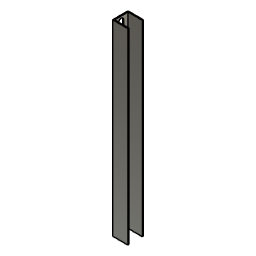
strut v1 (Autodesk Fusion 360 design; units mm, degrees)
Autodesk Fusion 360 part; units mm, degrees
sketch "Sketch1" plane through (0, 0, 0) normal (0, 0, 1) x (1, 0, 0)
  line L0 (20.5, 20.5) -> (-20.5, 20.5)
  line L1 (-20.5, 20.5) -> (-20.5, -20.5)
  line L2 (-20.5, -20.5) -> (20.5, -20.5)
  line L3 (20.5, -20.5) -> (20.5, 20.5)
  line L4 (20.5, 20.5) -> (-20.5, -20.5) construction
  line L5 (-20.5, 20.5) -> (20.5, -20.5) construction
  line L6 (-18, -18) -> (18, -18)
  line L7 (18, -18) -> (18, 18)
  line L8 (18, 18) -> (-18, 18)
  line L9 (-18, 18) -> (-18, -18)
  line L10 (18, 18) -> (20.5, 18)
  line L11 (20.5, 18) -> (20.5, -18)
  line L12 (20.5, -18) -> (18, -18)
  line L13 (18, -18) -> (18, 18)
  dimension "d1" = 41
  dimension "d2" = 41
  dimension "d3" = -2.5
  constraint horizontal L0
  constraint perpendicular L0 L1
  constraint parallel L0 L2
  constraint parallel L1 L3
  constraint coincident L4 origin
  constraint coincident L5 origin
  constraint horizontal L10
  constraint vertical L11
  constraint horizontal L12
  constraint vertical L13
  constraint coincident L3 L11.end
  measures "d1" distance of L1.end L2.end
  measures "d2" distance of L0.end L1.end
extrude "Extrude1" add sketch "Sketch1" along normal blind 500 contours L0 L1 L2 L3 L6 L8 L9 L10 L12
sketch "Sketch2" plane through (-20.5, 0, 0) normal (-1, 0, 0) x (0, -1, 0)
  line L0 (-20.5, 0) -> (20.5, 0)
  line L1 (20.5, 0) -> (20.5, 500)
  line L2 (20.5, 500) -> (-20.5, 500)
  line L3 (-20.5, 500) -> (-20.5, 0)
  line L4 (0, 500) -> (0, 495)
  line L5 (-6.5, 488.5) -> (-6.5, 461.5)
  line L6 (6.5, 488.5) -> (6.5, 461.5)
  arc A0 (0, 495) -> (-6.5, 488.5) centre (0, 488.5) ccw
  arc A1 (-6.5, 461.5) -> (0, 455) centre (0, 461.5) ccw
  arc A2 (0, 455) -> (6.5, 461.5) centre (0, 461.5) ccw
  arc A3 (6.5, 488.5) -> (0, 495) centre (0, 488.5) ccw
  line L7 (0, 455) -> (0, 432.5)
  line L8 (-6.5, 426) -> (-6.5, 399)
  arc A4 (0, 432.5) -> (-6.5, 426) centre (0, 426) ccw
  arc A5 (6.5, 426) -> (0, 432.5) centre (0, 426) ccw
  line L9 (6.5, 426) -> (6.5, 399)
  arc A6 (0, 392.5) -> (6.5, 399) centre (0, 399) ccw
  arc A7 (-6.5, 399) -> (0, 392.5) centre (0, 399) ccw
  line L10 (-6.5, 363.5) -> (-6.5, 336.5)
  arc A8 (0, 370) -> (-6.5, 363.5) centre (0, 363.5) ccw
  arc A9 (6.5, 363.5) -> (0, 370) centre (0, 363.5) ccw
  line L11 (6.5, 363.5) -> (6.5, 336.5)
  arc A10 (0, 330) -> (6.5, 336.5) centre (0, 336.5) ccw
  arc A11 (-6.5, 336.5) -> (0, 330) centre (0, 336.5) ccw
  line L12 (-6.5, 301) -> (-6.5, 274)
  arc A12 (0, 307.5) -> (-6.5, 301) centre (0, 301) ccw
  arc A13 (6.5, 301) -> (0, 307.5) centre (0, 301) ccw
  line L13 (6.5, 301) -> (6.5, 274)
  arc A14 (0, 267.5) -> (6.5, 274) centre (0, 274) ccw
  arc A15 (-6.5, 274) -> (0, 267.5) centre (0, 274) ccw
  line L14 (-6.5, 238.5) -> (-6.5, 211.5)
  arc A16 (0, 245) -> (-6.5, 238.5) centre (0, 238.5) ccw
  arc A17 (6.5, 238.5) -> (0, 245) centre (0, 238.5) ccw
  line L15 (6.5, 238.5) -> (6.5, 211.5)
  arc A18 (0, 205) -> (6.5, 211.5) centre (0, 211.5) ccw
  arc A19 (-6.5, 211.5) -> (0, 205) centre (0, 211.5) ccw
  line L16 (-6.5, 176) -> (-6.5, 149)
  arc A20 (0, 182.5) -> (-6.5, 176) centre (0, 176) ccw
  arc A21 (6.5, 176) -> (0, 182.5) centre (0, 176) ccw
  line L17 (6.5, 176) -> (6.5, 149)
  arc A22 (0, 142.5) -> (6.5, 149) centre (0, 149) ccw
  arc A23 (-6.5, 149) -> (0, 142.5) centre (0, 149) ccw
  line L18 (-6.5, 113.5) -> (-6.5, 86.5)
  arc A24 (0, 120) -> (-6.5, 113.5) centre (0, 113.5) ccw
  arc A25 (6.5, 113.5) -> (0, 120) centre (0, 113.5) ccw
  line L19 (6.5, 113.5) -> (6.5, 86.5)
  arc A26 (0, 80) -> (6.5, 86.5) centre (0, 86.5) ccw
  arc A27 (-6.5, 86.5) -> (0, 80) centre (0, 86.5) ccw
  line L20 (-6.5, 51) -> (-6.5, 24)
  arc A28 (0, 57.5) -> (-6.5, 51) centre (0, 51) ccw
  arc A29 (6.5, 51) -> (0, 57.5) centre (0, 51) ccw
  line L21 (6.5, 51) -> (6.5, 24)
  arc A30 (0, 17.5) -> (6.5, 24) centre (0, 24) ccw
  arc A31 (-6.5, 24) -> (0, 17.5) centre (0, 24) ccw
  point P0 (-6.5, 495)
  dimension "d6" = 5
  dimension "d7" = 6.5
  dimension "d10" = 6.5
  dimension "d11" = 22.5
  dimension "d14" = 0
  dimension "d15" = -62.5
  constraint midpoint L2 L4.start
  constraint perpendicular L2 L4
  constraint vertical L5
  constraint vertical L6
  constraint coincident P0 L5
  constraint tangent L5 A0
  constraint coincident L4.end A0.start
  constraint tangent L5 A1
  constraint equal A0 A1
  constraint tangent L6 A2
  constraint equal A0 A2
  constraint tangent L6 A3
  constraint equal A0 A3
  constraint parallel L6 L7
  measures "d6" distance of L4.start L4.end
  measures "d7" distance of L4.end P0
  measures "d10" radius of A0
  measures "d11" distance of A1.end L7.end
extrude "Extrude2" cut sketch "Sketch2" against normal blind 19.782 contours L5 L6 A0 A1 A2 A3 | L8 A4 A5 L9 A6 A7 | L10 A8 A9 L11 A10 A11 | L12 A12 A13 L13 A14 A15 | L14 A16 A17 L15 A18 A19 | L16 A20 A21 L17 A22 A23 | L18 A24 A25 L19 A26 A27 | L20 A28 A29 L21 A30 A31
equation "d7 = ( 13 / 2 ) * 1 mm"
equation "d10 = ( 13 / 2 ) * 1 mm"
